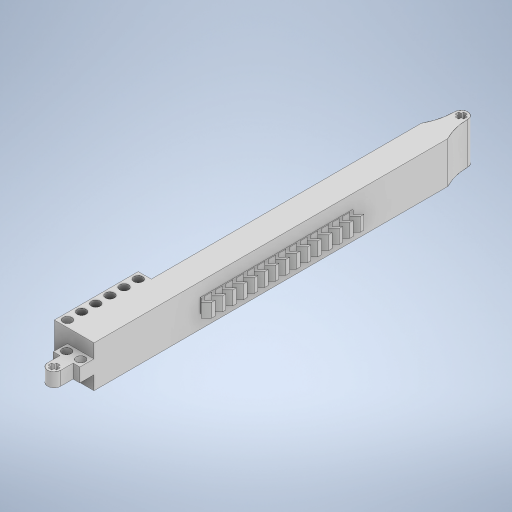
# Autodesk Inventor part: ramiev4
Saved by Autodesk Inventor 2023 (Build 270158000, 158)
## iProperties
Created: 2022-10-20
Part Number: ramiev4
Material: Ogólny
Document SubType Name: Modeling
Designer: kamil
Density: 1 g/cm^3
Appearance: Domyślna
Author: kamil
Autodesk Inventor part; units mm, degrees
ref_plane "YZ Plane" through (0, 0, 0) normal (1, 0, 0) x (0, 1, 0)
ref_plane "XZ Plane" through (0, 0, 0) normal (0, 1, 0) x (-1, 0, 0)
ref_plane "XY Plane" through (0, 0, 0) normal (0, 0, 1) x (1, 0, 0)
sketch "Sketch2" plane through (0, 0, 0) normal (0, 1, 0) x (-1, 0, 0)
  line L0 (7.5, 215) -> (-7.5, 215)
  line L1 (-7.5, 215) -> (-7.5, 15)
  line L2 (-7.5, 15) -> (7.5, 15)
  line L3 (7.5, 15) -> (7.5, 215)
  circle A0 centre (0, 0) radius 3.7
  line L4 (0, 215) -> (0, 15) construction
  line L5 (7.5, 215) -> (14.9, 215)
  line L6 (14.9, 215) -> (14.9, 167.6)
  line L7 (14.9, 167.6) -> (7.5, 167.6)
  line L8 (7.5, 167.6) -> (7.5, 215)
  arc A1 (7.5, 15) -> (3.7, 0) centre (35.2053, 0) ccw
  arc A2 (-3.7, 0) -> (-7.5, 15) centre (-35.2053, 0) ccw
  circle A3 centre (11.2, 171.3) radius 2.5
  circle A4 centre (11.2, 179.3) radius 2.5
  circle A5 centre (11.2, 187.3) radius 2.5
  circle A6 centre (11.2, 195.3) radius 2.5
  circle A7 centre (11.2, 203.3) radius 2.5
  circle A8 centre (11.2, 211.3) radius 2.5
  line L9 (-8, 117) -> (-10, 119)
  line L10 (-10, 119) -> (-12, 117)
  line L11 (-12, 117) -> (-13, 118) construction
  line L12 (-13, 118) -> (-10, 121)
  line L13 (-10, 121) -> (-8, 119)
  line L14 (-13, 118) -> (-13, 116)
  line L15 (-13, 116) -> (-12, 117)
  line L16 (-7.5, 155) -> (-8, 155)
  line L17 (-8, 155) -> (-8, 69)
  line L18 (-8, 69) -> (-7.5, 69)
  line L19 (-7.5, 69) -> (-7.5, 155)
  line L20 (-8, 119) -> (-8, 117)
  line L21 (-8, 153) -> (-10, 155)
  line L22 (-10, 155) -> (-12, 153)
  line L23 (-13, 154) -> (-10, 157)
  line L24 (-12, 153) -> (-13, 154) construction
  line L25 (-13, 154) -> (-13, 152)
  line L26 (-13, 152) -> (-12, 153)
  line L27 (-10, 157) -> (-8, 155)
  line L28 (-8, 155) -> (-8, 153)
  line L29 (-8, 147) -> (-10, 149)
  line L30 (-10, 149) -> (-12, 147)
  line L31 (-13, 148) -> (-10, 151)
  line L32 (-12, 147) -> (-13, 148) construction
  line L33 (-13, 148) -> (-13, 146)
  line L34 (-13, 146) -> (-12, 147)
  line L35 (-10, 151) -> (-8, 149)
  line L36 (-8, 149) -> (-8, 147)
  line L37 (-8, 141) -> (-10, 143)
  line L38 (-10, 143) -> (-12, 141)
  line L39 (-13, 142) -> (-10, 145)
  line L40 (-12, 141) -> (-13, 142) construction
  line L41 (-13, 142) -> (-13, 140)
  line L42 (-13, 140) -> (-12, 141)
  line L43 (-10, 145) -> (-8, 143)
  line L44 (-8, 143) -> (-8, 141)
  line L45 (-8, 135) -> (-10, 137)
  line L46 (-10, 137) -> (-12, 135)
  line L47 (-13, 136) -> (-10, 139)
  line L48 (-12, 135) -> (-13, 136) construction
  line L49 (-13, 136) -> (-13, 134)
  line L50 (-13, 134) -> (-12, 135)
  line L51 (-10, 139) -> (-8, 137)
  line L52 (-8, 137) -> (-8, 135)
  line L53 (-8, 129) -> (-10, 131)
  line L54 (-10, 131) -> (-12, 129)
  line L55 (-13, 130) -> (-10, 133)
  line L56 (-12, 129) -> (-13, 130) construction
  line L57 (-13, 130) -> (-13, 128)
  line L58 (-13, 128) -> (-12, 129)
  line L59 (-10, 133) -> (-8, 131)
  line L60 (-8, 131) -> (-8, 129)
  line L61 (-8, 123) -> (-10, 125)
  line L62 (-10, 125) -> (-12, 123)
  line L63 (-13, 124) -> (-10, 127)
  line L64 (-12, 123) -> (-13, 124) construction
  line L65 (-13, 124) -> (-13, 122)
  line L66 (-13, 122) -> (-12, 123)
  line L67 (-10, 127) -> (-8, 125)
  line L68 (-8, 125) -> (-8, 123)
  line L69 (-8, 111) -> (-10, 113)
  line L70 (-10, 113) -> (-12, 111)
  line L71 (-13, 112) -> (-10, 115)
  line L72 (-12, 111) -> (-13, 112) construction
  line L73 (-13, 112) -> (-13, 110)
  line L74 (-13, 110) -> (-12, 111)
  line L75 (-10, 115) -> (-8, 113)
  line L76 (2.4, 1.05) -> (-2.4, 1.05)
  line L77 (-2.4, 1.05) -> (-2.4, -1.05)
  line L78 (-2.4, -1.05) -> (2.4, -1.05)
  line L79 (2.4, -1.05) -> (2.4, 1.05)
  line L80 (1.05, 2.4) -> (-1.05, 2.4)
  line L81 (-1.05, 2.4) -> (-1.05, -2.4)
  line L82 (-1.05, -2.4) -> (1.05, -2.4)
  line L83 (1.05, -2.4) -> (1.05, 2.4)
  line L84 (7.5, 215) -> (-7.5, 215)
  circle A9 centre (0, 230) radius 3.7
  line L85 (-2.4, 228.95) -> (2.4, 228.95)
  line L86 (2.4, 228.95) -> (2.4, 231.05)
  line L87 (2.4, 231.05) -> (-2.4, 231.05)
  line L88 (-2.4, 231.05) -> (-2.4, 228.95)
  line L89 (-1.05, 227.6) -> (1.05, 227.6)
  line L90 (1.05, 227.6) -> (1.05, 232.4)
  line L91 (1.05, 232.4) -> (-1.05, 232.4)
  line L92 (-1.05, 232.4) -> (-1.05, 227.6)
  line L93 (0, 232.4) -> (0, 227.6) construction
  line L94 (3.7, 230) -> (3.7, 223)
  line L95 (3.7, 223) -> (7.5, 223)
  line L96 (7.5, 223) -> (7.5, 215)
  line L97 (-3.7, 230) -> (-3.7, 223)
  line L98 (-3.7, 223) -> (-7.5, 223)
  line L99 (-7.5, 223) -> (-7.5, 215)
  circle A10 centre (-4, 219) radius 2.5
  circle A11 centre (4, 219) radius 2.5
  line L100 (-13, 106) -> (-10, 109)
  line L101 (-8, 105) -> (-10, 107)
  line L102 (-10, 107) -> (-12, 105)
  line L103 (-12, 105) -> (-13, 106) construction
  line L104 (-13, 104) -> (-12, 105)
  line L105 (-13, 106) -> (-13, 104)
  line L106 (-10, 109) -> (-8, 107)
  line L107 (-13, 100) -> (-10, 103)
  line L108 (-8, 99) -> (-10, 101)
  line L109 (-10, 101) -> (-12, 99)
  line L110 (-12, 99) -> (-13, 100) construction
  line L111 (-13, 98) -> (-12, 99)
  line L112 (-13, 100) -> (-13, 98)
  line L113 (-10, 103) -> (-8, 101)
  line L114 (-13, 94) -> (-10, 97)
  line L115 (-8, 93) -> (-10, 95)
  line L116 (-10, 95) -> (-12, 93)
  line L117 (-12, 93) -> (-13, 94) construction
  line L118 (-13, 92) -> (-12, 93)
  line L119 (-13, 94) -> (-13, 92)
  line L120 (-10, 97) -> (-8, 95)
  line L121 (-13, 88) -> (-10, 91)
  line L122 (-8, 87) -> (-10, 89)
  line L123 (-10, 89) -> (-12, 87)
  line L124 (-12, 87) -> (-13, 88) construction
  line L125 (-13, 86) -> (-12, 87)
  line L126 (-13, 88) -> (-13, 86)
  line L127 (-10, 91) -> (-8, 89)
  line L128 (-13, 82) -> (-10, 85)
  line L129 (-8, 81) -> (-10, 83)
  line L130 (-10, 83) -> (-12, 81)
  line L131 (-12, 81) -> (-13, 82) construction
  line L132 (-13, 80) -> (-12, 81)
  line L133 (-13, 82) -> (-13, 80)
  line L134 (-10, 85) -> (-8, 83)
  line L135 (-13, 76) -> (-10, 79)
  line L136 (-8, 75) -> (-10, 77)
  line L137 (-10, 77) -> (-12, 75)
  line L138 (-12, 75) -> (-13, 76) construction
  line L139 (-13, 74) -> (-12, 75)
  line L140 (-13, 76) -> (-13, 74)
  line L141 (-10, 79) -> (-8, 77)
  line L142 (-13, 70) -> (-10, 73)
  line L143 (-8, 69) -> (-10, 71)
  line L144 (-10, 71) -> (-12, 69)
  line L145 (-12, 69) -> (-13, 70) construction
  line L146 (-13, 68) -> (-12, 69)
  line L147 (-13, 70) -> (-13, 68)
  line L148 (-10, 73) -> (-8, 71)
  point P0 (7.5, 115)
  point P1 (0, 115)
  point P2 (11.2, 167.6)
  point P3 (2.4, 0)
  point P4 (1.05, 0)
  point P5 (0, 2.4)
  point P6 (0, 1.05)
  point P7 (0, 147.3448)
  point P8 (-2.4, 230)
  point P9 (-1.05, 230)
  point P10 (0, 228.95)
  point P11 (0, 215)
  point P12 (2.4, 230)
  point P13 (-1.05, 1.05)
  point P14 (1.05, 1.05)
  point P15 (1.05, -1.05)
  point P16 (-1.05, -1.05)
  point P17 (7.5, 167.6)
  point P18 (-8, 153)
  point P19 (-8, 147)
  point P20 (-8, 141)
  point P21 (-8, 135)
  point P22 (-8, 129)
  point P23 (-8, 123)
  point P24 (-8, 117)
  point P25 (-8, 111)
  point P26 (-7.5, 69)
  point P27 (1.05, 228.95)
  point P28 (-1.05, 228.95)
  point P29 (-1.05, 231.05)
  point P30 (1.05, 231.05)
  dimension "d6" = 7.4
  dimension "d7" = 15
  dimension "d9" = 200
  dimension "d10" = 7.4
  dimension "d11" = 15
  dimension "d12" = 47.4
  dimension "d13" = 5
  dimension "d14" = 3.7
  dimension "d15" = 5
  dimension "d16" = 8
  dimension "d17" = 5
  dimension "d18" = 5
  dimension "d19" = 8
  dimension "d20" = 5
  dimension "d21" = 5
  dimension "d22" = 8
  dimension "d23" = 8
  dimension "d24" = 8
  dimension "d31" = 2
  dimension "d41" = 0.5
  dimension "d42" = 60
  dimension "d43" = 86
  dimension "d44" = 2
  dimension "d47" = 5
  dimension "d48" = 2
  dimension "d49" = 2
  dimension "d50" = 5
  dimension "d51" = 2
  dimension "d52" = 2
  dimension "d53" = 5
  dimension "d54" = 2
  dimension "d55" = 2
  dimension "d56" = 5
  dimension "d57" = 2
  dimension "d58" = 2
  dimension "d59" = 5
  dimension "d60" = 6
  dimension "d62" = 6
  dimension "d63" = 6
  dimension "d64" = 2
  dimension "d65" = 2
  dimension "d66" = 5
  dimension "d67" = 2
  dimension "d68" = 2
  dimension "d69" = 5
  dimension "d70" = 6
  dimension "d71" = 6
  dimension "d72" = 6
  dimension "d73" = 2
  dimension "d74" = 2
  dimension "d75" = 5
  dimension "d76" = 6
  dimension "d77" = 2.1
  dimension "d79" = 4.8
  dimension "d80" = 2.1
  dimension "d81" = 4.8
  dimension "d82" = 7.4
  dimension "d83" = 15
  dimension "d85" = 2.1
  dimension "d86" = 4.8
  dimension "d87" = 2.1
  dimension "d88" = 4.8
  dimension "d89" = 15
  dimension "d92" = 5
  constraints: 296 end point, 44 perpendicular, 29 vertical alignment, 20 vertical, 17 midpoint, 13 horizontal alignment, 13 parallel, 12 centre point, 8 collinear, 8 point on circle, 6 horizontal, 3 coincident, 3 tangent, 1 point on line, 110 other
  measures "d6" diameter of A0
  measures "d7" distance of L1.end L2.end
  measures "d9" distance of L2.end L0.start
  measures "d10" distance of L6.end L7.end
  measures "d11" distance of A0.centre L4.end
  measures "d12" distance of L5.end L6.end
  measures "d13" diameter of A3
  measures "d14" distance of point (11.2, 167.6) A3.centre
  measures "d15" diameter of A4
  measures "d16" distance of A4.centre A3.centre
  measures "d17" diameter of A5
  measures "d18" diameter of A6
  measures "d19" distance of A6.centre A5.centre
  measures "d20" diameter of A7
  measures "d21" diameter of A8
  measures "d22" distance of A8.centre A7.centre
  measures "d23" distance of A6.centre A7.centre
  measures "d24" distance of A4.centre A5.centre
  measures "d31" distance of L12.end L9.end
  measures "d41" distance of L18.start L18.end
  measures "d42" distance of L0.end L16.start
  measures "d43" distance of L18.end L16.start
  measures "d44" distance of L9.end L13.end
  measures "d47" horizontal distance of L14.end L9.start
  measures "d48" distance of L27.start L21.end
  measures "d49" distance of L16.end L21.end
  measures "d50" horizontal distance of L25.end L28.end
  measures "d51" distance of L35.start L29.end
  measures "d52" distance of L29.end L36.start
  measures "d53" horizontal distance of L33.end L36.end
  measures "d54" distance of L43.start L37.end
  measures "d55" distance of L37.end L44.start
  measures "d56" horizontal distance of L41.end L44.end
  measures "d57" distance of L51.start L45.end
  measures "d58" distance of L45.end L52.start
  measures "d59" horizontal distance of L49.end L52.end
  measures "d60" distance of L36.end L28.end
  measures "d62" distance of L44.end L36.end
  measures "d63" distance of L52.end L44.end
  measures "d64" distance of L59.start L53.end
  measures "d65" distance of L53.end L60.start
  measures "d66" horizontal distance of L57.end L60.end
  measures "d67" distance of L67.start L61.end
  measures "d68" distance of L61.end L68.start
  measures "d69" horizontal distance of L65.end L68.end
  measures "d70" distance of L60.end L52.end
  measures "d71" distance of L68.end L60.end
  measures "d72" distance of L9.start L68.end
  measures "d73" distance of L75.start L70.start
  measures "d74" distance of L70.start L75.end
  measures "d75" horizontal distance of L74.start L69.start
  measures "d76" distance of L9.start L69.start
  measures "d77" distance of L81.end L82.end
  measures "d79" distance of L82.end L80.start
  measures "d80" distance of L78.end L76.start
  measures "d81" distance of L77.end L78.end
  measures "d82" diameter of A9
  measures "d83" distance of L0.start L84.end
  measures "d85" distance of L90.end L91.end
  measures "d86" distance of L91.end L89.start
  measures "d87" distance of L87.end L85.start
  measures "d88" distance of L86.end L87.end
  measures "d89" vertical distance of L0.start A9.centre
  measures "d92" diameter of A10
extrude "Extrusion1" add sketch "Sketch2" along normal blind 23.4 contours L3 L2 L1 L0 | L5 L6 L7 L3 | A1 A0 A2 L2 | A0
extrude "Extrusion2" add sketch "Sketch2" along normal blind 15.6 contours L0 L99 L98 L97 A9 L94 L95 L96 | L1 L18 L17 L16 | L17 L21 L22 L26 L25 L23 L27 | A9 | L143 L144 L146 L147 L142 L148 L17 | L17 L29 L30 L34 L33 L31 L35 | L136 L137 L139 L140 L135 L141 L17 | L17 L37 L38 L42 L41 L39 L43 | L129 L130 L132 L133 L128 L134 L17 | L17 L45 L46 L50 L49 L47 L51 | L122 L123 L125 L126 L121 L127 L17 | L17 L53 L54 L58 L57 L55 L59 | L115 L116 L118 L119 L114 L120 L17 | L17 L61 L62 L66 L65 L63 L67 | L108 L109 L111 L112 L107 L113 L17 | L17 L9 L10 L15 L14 L12 L13 | L101 L102 L104 L105 L100 L106 L17 | L17 L69 L70 L74 L73 L71 L75
extrude "Extrusion3" cut sketch "Sketch2" along normal blind 7.8 contours L0 L99 L98 L97 A9 L94 L95 L96 | L1 L18 L17 L16 | L17 L21 L22 L26 L25 L23 L27 | A9 | L143 L144 L146 L147 L142 L148 L17 | L17 L29 L30 L34 L33 L31 L35 | L136 L137 L139 L140 L135 L141 L17 | L17 L37 L38 L42 L41 L39 L43 | L129 L130 L132 L133 L128 L134 L17 | L17 L45 L46 L50 L49 L47 L51 | L122 L123 L125 L126 L121 L127 L17 | L17 L53 L54 L58 L57 L55 L59 | L115 L116 L118 L119 L114 L120 L17 | L17 L61 L62 L66 L65 L63 L67 | L108 L109 L111 L112 L107 L113 L17 | L17 L9 L10 L15 L14 L12 L13 | L101 L102 L104 L105 L100 L106 L17 | L17 L69 L70 L74 L73 L71 L75
equation "\"d10\" = d6"
equation "\"d14\" = 0.5 * d6"
equation "\"d15\" = d13"
equation "\"d18\" = d17"
equation "\"d21\" = d20"
equation "\"d23\" = d16"
equation "\"d24\" = d16"
body "Solid3"
